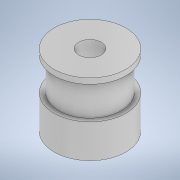
# Autodesk Inventor part: Gt2_20_5
Saved by Autodesk Inventor 2021 (Build 250183000, 183)
## iProperties
Created: 2021-04-05
Part Number: Gt2_20_5
Material: Generic
Document SubType Name: Modeling
Designer: jorge
Density: 1 g/cm^3
Appearance: Aluminum - Polished
Author: jorge
Autodesk Inventor part; units mm, degrees
ref_plane "YZ Plane" through (0, 0, 0) normal (1, 0, 0) x (0, 1, 0)
ref_plane "XZ Plane" through (0, 0, 0) normal (0, 1, 0) x (-1, 0, 0)
sketch "Sketch1" plane through (0, 0, 0) normal (0, 1, 0) x (-1, 0, 0)
  circle A0 centre (0, 0) radius 8
  circle A1 centre (0, 0) radius 2.5
  dimension "d0" = 16
  dimension "d1" = 5
  constraints: 2 centre point, 2 coincident
  measures "d0" diameter of A0
  measures "d1" diameter of A1
extrude "Extrusion1" add sketch "Sketch1" along normal blind 16
ref_plane "Work Plane1" through (0, 14.75, 0) normal (0, 1, 0) x (1, 0, 0)
sketch "Sketch2" plane through (0, 14.75, 0) normal (0, 1, 0) x (1, 0, 0)
  circle A0 centre (0, 0) radius 8
  circle A1 centre (0, 0) radius 8 projected
  circle A2 centre (0, 0) radius 7
  dimension "d5" = 1
  constraints: 2 centre point, 1 coincident, 1 concentric
  measures "d5" radial gap between concentric circles of A0 A2
extrude "Extrusion2" cut sketch "Sketch2" against normal blind 7.25
body "Solid1"
